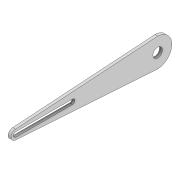
# Autodesk Inventor part: CorrederaPalanca
Saved by Autodesk Inventor 2021 (Build 250183000, 183)
## iProperties
Created: 2021-05-09
Part Number: CorrederaPalanca
Material: Genérico
Document SubType Name: Modeling
Designer: carlo
Density: 1 g/cm^3
Appearance: Valor por defecto
Author: carlo
Autodesk Inventor part; units mm, degrees
ref_plane "YZ Plane" through (0, 0, 0) normal (1, 0, 0) x (0, 1, 0)
ref_plane "XZ Plane" through (0, 0, 0) normal (0, 1, 0) x (-1, 0, 0)
ref_plane "XY Plane" through (0, 0, 0) normal (0, 0, 1) x (1, 0, 0)
sketch "Boceto1" plane through (0, 30.6548, -58.1067) normal (1, 0, 0) x (0, 1, 0)
  arc A0 (-13.6856, -6.1404) -> (15, 0) centre (0, 0) ccw
  arc A1 (-13.6856, -6.1404) -> (14.8675, 1.989) centre (0, 0) ccw
  arc A2 (-13.6856, -6.1404) -> (15, 0) centre (0, 0) ccw
  circle A3 centre (0, 0) radius 5
  arc A4 (-14.8673, 1.9912) -> (14.8675, 1.989) centre (0, 0) ccw
  arc A5 (-2.5, 90) -> (2.5, 90) centre (0, 90) ccw
  arc A6 (2.5, 150) -> (-2.5, 150) centre (0, 150) ccw
  line L0 (2.5, 150) -> (2.5, 90)
  line L1 (-2.5, 150) -> (-2.5, 90)
  line L2 (15, 0) -> (4.989, 150.3322)
  line L3 (-15, 0) -> (-5, 150)
  arc A7 (4.989, 150.3322) -> (-5, 150) centre (0, 150) ccw
  point P0 (15, 0)
  point P1 (15, 0)
  constraints: 16 point on circle, 8 centre point, 8 end point, 3 coincident, 2 point on line, 2 tangent, 1 vertical
extrude "Extrusión1" add sketch "Boceto1" along normal blind 3 contours A4 L3 A7 L2 A0
